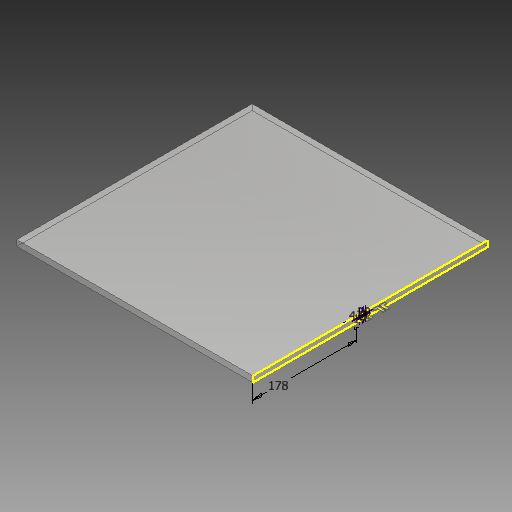
# Autodesk Inventor part: PV_Modul_CPY_3_CPY2
Saved by Autodesk Inventor 2018.3 (Build 223284000, 284)
## iProperties
Created: 2019-08-12
Part Number: PV_Modul_CPY_3_CPY2
Material: Glas
Document SubType Name: Modeling
Designer: DerLobre
Density: 2.18 g/cm^3
Appearance: Klar
Author: DerLobre
Autodesk Inventor part; units mm, degrees
ref_plane "YZ Plane" through (0, 0, 0) normal (1, 0, 0) x (0, 1, 0)
ref_plane "XZ Plane" through (0, 0, 0) normal (0, 1, 0) x (-1, 0, 0)
ref_plane "XY Plane" through (0, 0, 0) normal (0, 0, 1) x (1, 0, 0)
sketch "Skizze1" plane through (0, 0, 0) normal (0, 0, 1) x (1, 0, 0)
  line L0 (-200, 200) -> (200, 200)
  line L1 (200, 200) -> (200, -200)
  line L2 (200, -200) -> (-200, -200)
  line L3 (-200, -200) -> (-200, 200)
  line L4 (-280, 0) -> (280, 0) projected
  line L5 (0, -280) -> (0, 280) projected
  point P0 (0, 0)
  dimension "d0" = 400
  dimension "d1" = 400
  constraints: 8 end point, 2 parallel, 1 horizontal, 1 perpendicular, 2 other
  measures "d0" distance of L1.end L2.end
  measures "d1" distance of L0.end L1.end
extrude "Extrusion1" add sketch "Skizze1" along normal blind 10
sketch "Skizze2" plane through (200, -200, 0) normal (1, 0, 0) x (0, 0, -1)
  line L0 (0, 400) -> (0, 0) projected
  line L1 (0, 400) -> (-10, 400) projected
  line L2 (-10, 0) -> (-10, 400) projected
  line L3 (0, 0) -> (-10, 0) projected
  line L4 (-5.5, 182.5) -> (-4.5, 182.5)
  line L5 (-4.5, 182.5) -> (-4.5, 193.5)
  line L6 (-4.5, 193.5) -> (-5.5, 193.5)
  line L7 (-5.5, 193.5) -> (-5.5, 182.5)
  line L8 (-5.5, 182.5) -> (-4.5, 182.5)
  line L9 (-4.5, 182.5) -> (-4.5, 187)
  line L10 (-4.5, 187) -> (-5.5, 187)
  line L11 (-5.5, 187) -> (-5.5, 182.5)
  line L12 (-5.5, 189) -> (-4.5, 189)
  line L13 (-4.5, 189) -> (-4.5, 193.5)
  line L14 (-4.5, 193.5) -> (-5.5, 193.5)
  line L15 (-5.5, 193.5) -> (-5.5, 189)
  line L16 (-5.5, 182.5) -> (-4.5, 182.5)
  line L17 (-4.5, 182.5) -> (-4.5, 178)
  line L18 (-4.5, 178) -> (-5.5, 178)
  line L19 (-5.5, 178) -> (-5.5, 182.5)
  line L20 (-5.5, 193.5) -> (-4.5, 193.5)
  line L21 (-4.5, 193.5) -> (-4.5, 198)
  line L22 (-4.5, 198) -> (-5.5, 198)
  line L23 (-5.5, 198) -> (-5.5, 193.5)
  line L24 (-6.1285, 188) -> (-3.7092, 188)
  line L25 (-10, 0) -> (-10, 400) projected
  line L26 (0, 400) -> (0, 0) projected
  point P0 (0, 200)
  dimension "d4" = 20
  dimension "d5" = 1
  dimension "d6" = 11
  dimension "d7" = 2
  dimension "d8" = 4.5
  dimension "d10" = 178
  constraints: 42 end point, 13 parallel, 8 coincident, 6 horizontal, 5 perpendicular, 3 point on line, 3 other
  measures "d4" distance between parallel lines of L22 L18
  measures "d5" distance of L17.end L18.end
  measures "d6" distance between parallel lines of L6 L4
  measures "d7" distance between parallel lines of L12 L10
  measures "d8" distance between parallel lines of L25 L19
  measures "d10" distance from line of L3 L17.end
extrude "Extrusion2" add sketch "Skizze2" along normal blind 4 contours L7 L10 L5 L4 | L4 L17 L18 L19 | L7 L6 L5 L12 | L23 L22 L21 L6
extrude "Extrusion4" add sketch "Skizze2" along normal blind 13 contours L7 L10 L5 L4 | L7 L6 L5 L12
pattern_linear "Rechteckige Anordnung1" count 2 spacing 27 along (0, 1, 0) of "Extrusion4", "Extrusion2"
